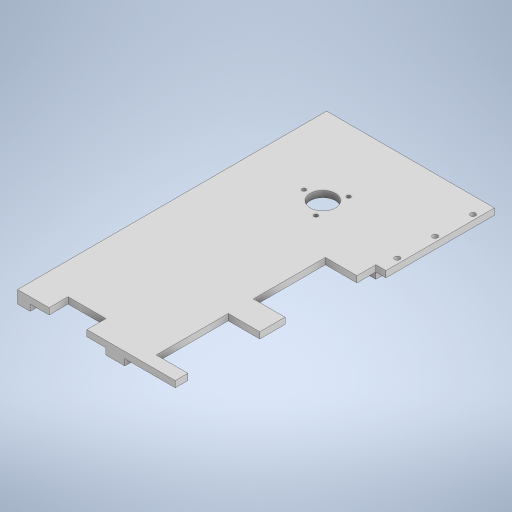
# Autodesk Inventor part: top_2
Saved by Autodesk Inventor 2023 (Build 270158000, 158)
## iProperties
Created: 2024-04-26
Part Number: top_2
Material: 常规
Document SubType Name: Modeling
Designer: Nitrene.P.L
Density: 1 g/cm^3
Appearance: 默认
Author: Nitrene.P.L
Autodesk Inventor part; units mm, degrees
ref_plane "YZ Plane" through (0, 0, 0) normal (1, 0, 0) x (0, 1, 0)
ref_plane "XZ Plane" through (0, 0, 0) normal (0, 1, 0) x (-1, 0, 0)
ref_plane "XY Plane" through (0, 0, 0) normal (0, 0, 1) x (1, 0, 0)
sketch "草图1" plane through (0, 0, 0) normal (0, 1, 0) x (-1, 0, 0)
  line L0 (125, 245) -> (-125, 245)
  line L1 (-125, 245) -> (-125, -245)
  line L2 (-125, -245) -> (125, -245)
  line L3 (125, -245) -> (125, 245)
  line L4 (0, 3) -> (0, -5)
  line L5 (3.5058, 0) -> (-3.4421, 0)
  line L6 (25, 144) -> (-32, 144)
  line L7 (-32, 144) -> (-32, 87)
  line L8 (-32, 87) -> (25, 87)
  line L9 (25, 87) -> (25, 144)
  line L10 (25, 67) -> (-32, 67)
  line L11 (-32, 67) -> (-32, 10)
  line L12 (-32, 10) -> (25, 10)
  line L13 (25, 10) -> (25, 67)
  line L14 (25, -10) -> (-32, -10)
  line L15 (-32, -10) -> (-32, -67)
  line L16 (-32, -67) -> (25, -67)
  line L17 (25, -67) -> (25, -10)
  line L18 (25, -87) -> (-32, -87)
  line L19 (-32, -87) -> (-32, -144)
  line L20 (-32, -144) -> (25, -144)
  line L21 (25, -144) -> (25, -87)
  line L22 (-66, 100) -> (-95, 100)
  line L23 (-95, 100) -> (-95, 54)
  line L24 (-95, 54) -> (-66, 54)
  line L25 (-66, 54) -> (-66, 100)
  line L26 (-66, -54) -> (-95, -54)
  line L27 (-95, -54) -> (-95, -100)
  line L28 (-95, -100) -> (-66, -100)
  line L29 (-66, -100) -> (-66, -54)
  line L30 (100, 15) -> (70, 15)
  line L31 (70, 15) -> (70, -15)
  line L32 (70, -15) -> (100, -15)
  line L33 (100, -15) -> (100, 15)
  circle A0 centre (65, 182) radius 10
  circle A1 centre (65, -182) radius 10
  circle A2 centre (65, 182) radius 15
  circle A3 centre (80, 182) radius 1.5
  circle A4 centre (57.5, 194.9904) radius 1.5
  circle A5 centre (57.5, 169.0096) radius 1.5
  line L34 (125, 245) -> (0, 245)
  line L35 (0, 245) -> (0, 0)
  line L36 (0, 0) -> (125, 0)
  line L37 (125, 0) -> (125, 245)
  line L38 (-125, 245) -> (0, 245)
  line L39 (0, 245) -> (0, 0)
  line L40 (0, 0) -> (-125, 0)
  line L41 (-125, 0) -> (-125, 245)
  line L42 (-125, -245) -> (0, -245)
  line L43 (0, -245) -> (0, 0)
  line L44 (0, 0) -> (-125, 0)
  line L45 (-125, 0) -> (-125, -245)
  line L46 (125, -245) -> (0, -245)
  line L47 (0, -245) -> (0, 0)
  line L48 (0, 0) -> (125, 0)
  line L49 (125, 0) -> (125, -245)
  circle A6 centre (65, -182) radius 15
  circle A7 centre (80, -182) radius 1.5
  circle A8 centre (57.5, -169.0096) radius 1.5
  circle A9 centre (57.5, -194.9904) radius 1.5
  point P0 (0, -144)
  point P1 (100, 0)
  point P2 (70, 0)
  point P3 (0, -10)
  point P4 (0, -67)
  point P5 (0, -87)
  dimension "d33" = 30
  dimension "d36" = 30
  dimension "d2" = 490
  dimension "d3" = 250
  dimension "d4" = 57
  dimension "d5" = 57
  dimension "d6" = 57
  dimension "d7" = 57
  dimension "d8" = 57
  dimension "d9" = 57
  dimension "d10" = 57
  dimension "d11" = 57
  dimension "d12" = 101
  dimension "d13" = 20
  dimension "d14" = 20
  dimension "d15" = 20
  dimension "d16" = 93
  dimension "d17" = 29
  dimension "d18" = 46
  dimension "d19" = 46
  dimension "d20" = 145
  dimension "d21" = 108
  dimension "d22" = 30
  dimension "d23" = 30
  dimension "d24" = 30
  dimension "d25" = 25
  dimension "d26" = 230
  dimension "d27" = 20
  dimension "d28" = 63
  dimension "d29" = 60
  dimension "d30" = 20
  dimension "d31" = 63
  dimension "d32" = 60
  dimension "d34" = 3
  dimension "d35" = 360
  dimension "d37" = 3
  dimension "d40" = 360
  constraints: 100 end point, 24 parallel, 14 horizontal, 12 perpendicular, 8 centre point, 3 collinear, 2 coincident, 2 horizontal alignment, 2 point on line, 2 vertical, 20 other
  measures "d2" distance of L3.start L3.end
  measures "d3" distance of L3.end L41.end
  measures "d4" distance of L8.end L7.end
  measures "d5" distance of L7.end L7.start
  measures "d6" distance of L12.end L11.end
  measures "d7" distance of L11.end L10.end
  measures "d8" distance of L16.end L15.end
  measures "d9" distance of L15.end L15.start
  measures "d10" distance of L20.end L19.end
  measures "d11" distance of L19.end L19.start
  measures "d12" distance between parallel lines of L0 L6
  measures "d13" distance between parallel lines of L10 L8
  measures "d14" distance between parallel lines of L12 L14
  measures "d15" distance between parallel lines of L18 L16
  measures "d16" distance between parallel lines of L1 L7
  measures "d17" distance of L24.end L24.start
  measures "d18" distance of L24.start L22.end
  measures "d19" distance of L27.end L27.start
  measures "d20" distance between parallel lines of L0 L22
  measures "d21" distance between parallel lines of L26 L24
  measures "d22" distance between parallel lines of L1 L23
  measures "d23" distance of L33.start L31.end
  measures "d24" distance of L31.end L30.end
  measures "d25" distance between parallel lines of L3 L33
  measures "d26" distance between parallel lines of L0 L30
  measures "d27" diameter of A0
  measures "d28" distance from line of L0 A0.centre
  measures "d29" distance from line of L3 A0.centre
  measures "d30" diameter of A1
  measures "d31" distance from line of L2 A1.centre
  measures "d32" distance from line of L3 A1.centre
  measures "d34" diameter of A3
  measures "d37" diameter of A7
extrude "拉伸1" add sketch "草图1" along normal blind 10 contours L3 L2 L43 L20 L21 L18 L16 L17 L14 L4 L5 L36 L31 L32 L33 | A7 A6 A9 A8
sketch "草图2" plane through (0, 0, 0) normal (0, -1, 0) x (1, 0, 0)
  line L0 (-70, 0) -> (0, 0) projected
  line L1 (-115, -30) -> (-55, -30)
  line L2 (-55, -30) -> (-55, 0)
  line L3 (-55, 0) -> (-115, 0)
  line L4 (-115, 0) -> (-115, -30)
  line L5 (-100, -15) -> (-70, -15) projected
  line L6 (-100, 0) -> (-100, -15) projected
  line L7 (-70, -15) -> (-70, 0) projected
  line L8 (-40, -159) -> (0, -159)
  line L9 (0, -159) -> (0, 0)
  line L10 (0, 0) -> (-40, 0)
  line L11 (-40, 0) -> (-40, -159)
  line L12 (-25, -10) -> (-25, -67) projected
  line L13 (-25, -144) -> (0, -144) projected
  circle A0 centre (-65, -182) radius 10 projected
  circle A1 centre (-65, -182) radius 20
  dimension "d44" = 15
  dimension "d45" = 15
  dimension "d46" = 15
  dimension "d47" = 15
  dimension "d48" = 15
  dimension "d49" = 40
  constraints: 16 end point, 4 parallel, 2 horizontal, 2 perpendicular, 1 centre point, 1 coincident, 1 point on line
  measures "d44" distance between parallel lines of L1 L5
  measures "d45" distance between parallel lines of L4 L6
  measures "d46" distance between parallel lines of L2 L7
  measures "d47" distance between parallel lines of L11 L12
  measures "d48" distance between parallel lines of L8 L13
  measures "d49" diameter of A1
extrude "拉伸2" cut sketch "草图2" against normal blind 5 contours L0 L2 L1 L4 L3 L6 L5 L7 | L0 L9 L8 L11 | A1
sketch "草图5" plane through (0, 10, 0) normal (0, 1, 0) x (1, 0, 0)
  line L0 (0, 159) -> (-40, 159) projected
  line L1 (0, 159) -> (8, 159)
  line L2 (8, 159) -> (8, 245)
  line L3 (8, 245) -> (0, 245)
  line L4 (0, 245) -> (0, 159)
  circle A0 centre (4, 172) radius 2
  circle A1 centre (4, 202) radius 2
  circle A2 centre (4, 232) radius 2
  point P0 (0, 0)
  dimension "d64" = 8
  dimension "d65" = 4
  dimension "d66" = 4
  dimension "d67" = 4
  dimension "d68" = 4
  dimension "d69" = 4
  dimension "d70" = 4
  dimension "d71" = 30
  dimension "d72" = 30
  dimension "d73" = 13
  constraints: 8 end point, 3 centre point, 2 parallel, 1 horizontal, 1 perpendicular
  measures "d64" distance of L3.end L2.end
  measures "d65" diameter of A0
  measures "d66" diameter of A1
  measures "d67" diameter of A2
  measures "d68" distance from line of L4 A0.centre
  measures "d69" distance from line of L4 A1.centre
  measures "d70" distance from line of L4 A2.centre
  measures "d71" distance of A1.centre A0.centre
  measures "d72" distance of A2.centre A1.centre
  measures "d73" distance from line of L1 A0.centre
extrude "拉伸4" add sketch "草图5" against normal blind 5
